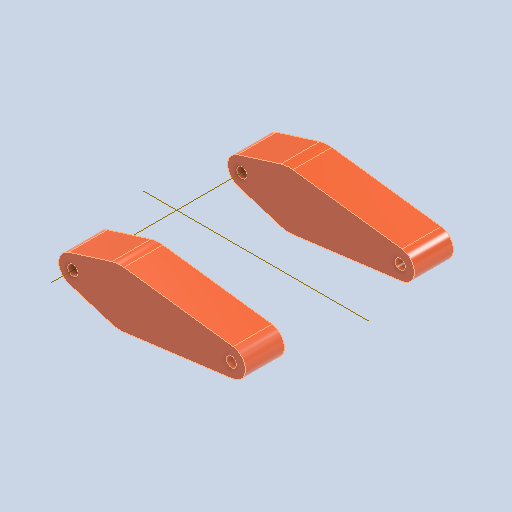
# Autodesk Inventor part: Type 1A R5主滑台連接桿:1
Saved by Autodesk Inventor 2025 (Build 290162000, 162)
## iProperties
Created: 2024-10-07
Part Number: Type 1A R5主滑台連接桿:1
Material: 密度7850的鋼
Document SubType Name: Modeling
Designer: user
Density: 7.84999 g/cm^3
Appearance: 平滑 - 淡橙色
Mass: 83102.8 g
Surface Area: 4644.6 cm^2
Volume: 10586.3 cm^3
Author: user
Autodesk Inventor part; units mm, degrees
ref_plane "YZ Plane" through (0, 0, 0) normal (1, 0, 0) x (0, 1, 0)
ref_plane "XZ Plane" through (0, 0, 0) normal (0, 1, 0) x (-1, 0, 0)
ref_plane "工作平面1" through (0, 0, 275) normal (0, 0, 1) x (1, 0, 0)
sketch "草圖1" plane through (0, 0, 275) normal (0, 0, 1) x (1, 0, 0)
  line L0 (0, 0) -> (419.3047, 0) construction
  arc A0 (-11.1792, 35.7949) -> (-11.1792, -35.7949) centre (0, 0) ccw
  arc A1 (424.0958, -37.1927) -> (424.0958, 37.1927) centre (419.3047, 0) ccw
  line L1 (-11.1792, -35.7949) -> (103.433, -71.5898)
  line L2 (135.3736, 74.3854) -> (424.0958, 37.1927)
  line L3 (-11.1792, 35.7949) -> (103.433, 71.5898)
  line L4 (135.3736, -74.3854) -> (424.0958, -37.1927)
  arc A2 (103.433, -71.5898) -> (135.3736, -74.3854) centre (125.7914, 0) ccw
  arc A3 (135.3736, 74.3854) -> (103.433, 71.5898) centre (125.7914, 0) ccw
  dimension "d3" = 419.3047
  dimension "d4" = 75
  dimension "d6" = 75
  dimension "d51" = 125.7914
  dimension "d52" = 75
  constraints: 10 end point, 8 point on circle, 8 tangent, 4 centre point, 2 coincident, 1 concentric, 1 horizontal, 1 point on line
  measures "d3" distance of L0.start L0.end
  measures "d4" diameter of A0
  measures "d6" diameter of A1
  measures "d51" distance of A2.centre L0.start
  measures "d52" radius of A3
extrude "擠出1" add sketch "草圖1" against normal blind 103
sketch "草圖2" plane through (0, 0, 275) normal (0, 0, 1) x (1, 0, 0)
  arc A0 (-11.1792, 35.7949) -> (-11.1792, -35.7949) centre (0, 0) ccw projected
  circle A1 centre (0, 0) radius 13.25
  arc A2 (424.0958, -37.1927) -> (424.0958, 37.1927) centre (419.3047, 0) ccw projected
  circle A3 centre (419.3047, 0) radius 13.25
  point P0 (-10.9663, -35.8607)
  point P1 (-34.5251, 14.6378)
  point P2 (141.4214, 141.4214)
  point P3 (444.0649, 33.6154)
  point P4 (432.144, -37.2043)
  dimension "d11" = 26.5
  dimension "d13" = 26.5
  constraints: 2 centre point, 2 coincident, 1 other
  measures "d11" diameter of A1
  measures "d13" diameter of A3
extrude "擠出2" cut sketch "草圖2" against normal through all
sketch "草圖3" plane through (434.4748, 35.8557, 275) normal (0.1277625, 0.9918048, 0) x (0.9918048, -0.1277625, 0)
  line L0 (-10.4648, 0) -> (-10.4648, 103) projected
  point P0 (-426.3332, 275)
  point P1 (-10.4648, 51.5)
  point P2 (-10.4648, 51.5)
  constraints: 1 coincident, 1 midpoint
hole "孔1" [suppressed]
sketch "草圖4" plane through (51.2031, 55.2777, 275) normal (-0.2981126, 0.9545307, 0) x (0.9545307, 0.2981126, 0)
  line L0 (-65.3539, 0) -> (-65.3539, 103) projected
  point P0 (-65.3539, 275)
  point P1 (-65.3539, 51.5)
  point P2 (-65.3539, 51.5)
  constraints: 1 coincident, 1 midpoint
hole "孔2" [suppressed]
sketch "草圖6" plane through (-11.1792, -35.7949, 172) normal (-0.2981126, -0.9545307, 0) x (0.9545307, -0.2981126, 0)
  line L0 (0, 51.5) -> (0, 0) projected
  point P0 (0, -172)
  point P1 (0, 25.75)
  constraints: 1 midpoint
hole "孔4" [suppressed]
sketch "草圖7" plane through (135.3736, -74.3854, 172) normal (0.1277625, -0.9918048, 0) x (0.9918048, 0.1277625, 0)
  line L0 (296.8516, 51.5) -> (296.8516, 0) projected
  point P0 (-124.7605, -172)
  point P1 (296.8516, 25.75)
  constraints: 1 midpoint
hole "孔5" [suppressed]
mirror "鏡射1" about plane through (0, 0, 0) normal (0, 0, 1) of "擠出1", "擠出2"
equation "\"d3\" = R5"
equation "\"d51\" = 0.3 * R5"
equation "\"R5\" = T1A_R5"
equation "\"th5a\" = T1A_th5a"
equation "\"d0\" = 0.5 * Width"
equation "\"T1A_R5\" = 419.3047"
equation "\"T1A_th5a\" = 45deg"
equation "\"T1A_R1\" = 585.5331"
equation "\"T1A_R3\" = 252.3048"
equation "\"T1A_R4\" = 320.6953"
equation "\"T1A_R7\" = -221.7475"
equation "\"T1A_R8\" = 369.2781"
equation "\"T1A_R1_Width\" = 756"
equation "\"T1A_R2_Width\" = 756"
equation "\"T1A_R3_Width\" = 344"
equation "\"T1A_R4_Width\" = 756"
equation "\"T1A_Joint_Width\" = 756"
equation "\"Width\" = 550"
